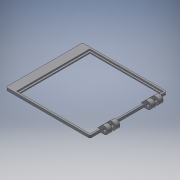
# Autodesk Inventor part: tampa acrilico
Saved by Autodesk Inventor 2019.4 (Build 234330000, 330)
## iProperties
Created: 2019-11-13
Part Number: tampa acrilico
Material: Genérico
Document SubType Name: Modeling
Designer: natha
Density: 1 g/cm^3
Appearance: Padrão
Author: natha
Autodesk Inventor part; units mm, degrees
ref_plane "YZ Plane" through (0, 0, 0) normal (1, 0, 0) x (0, 1, 0)
ref_plane "XZ Plane" through (0, 0, 0) normal (0, 1, 0) x (-1, 0, 0)
ref_plane "XY Plane" through (0, 0, 0) normal (0, 0, 1) x (1, 0, 0)
sketch "Esboço1" plane through (0, 0, 0) normal (0, 1, 0) x (-1, 0, 0)
  line L0 (-53, -48) -> (-53, 48)
  line L1 (-53, 48) -> (43, 48)
  line L2 (43, -48) -> (43, 48)
  line L3 (43, -48) -> (-53, -48)
  line L4 (-57, -52) -> (57, -52)
  line L5 (57, -52) -> (57, 52)
  line L6 (57, 52) -> (-57, 52)
  line L7 (-57, 52) -> (-57, 42.5)
  line L8 (-57, 42.5) -> (-57, 37.5)
  line L9 (-66.8204, 37.5) -> (-57, 37.5)
  line L10 (-66.8204, 31.9) -> (-66.8204, 37.5)
  line L11 (-66.8204, 31.9) -> (-57, 31.9)
  line L12 (-57, 31.9) -> (-57, 26.9)
  line L13 (-66.8204, 26.9) -> (-57, 26.9)
  line L14 (-66.8204, 21.3) -> (-66.8204, 26.9)
  line L15 (-66.8204, 21.3) -> (-57, 21.3)
  line L16 (-57, 21.3) -> (-57, 12.5)
  line L17 (-57, 12.5) -> (-57, -12.5)
  line L18 (-57, -12.5) -> (-57, -21.3)
  line L19 (-66.8204, -21.3) -> (-57, -21.3)
  line L20 (-66.8204, -26.9) -> (-66.8204, -21.3)
  line L21 (-66.8204, -26.9) -> (-57, -26.9)
  line L22 (-57, -26.9) -> (-57, -31.9)
  line L23 (-66.8204, -31.9) -> (-57, -31.9)
  line L24 (-66.8204, -37.5) -> (-66.8204, -31.9)
  line L25 (-66.8204, -37.5) -> (-57, -37.5)
  line L26 (-57, -37.5) -> (-57, -42.5)
  line L27 (-57, -42.5) -> (-57, -52)
  point P0 (0, 0)
  point P1 (0, 0)
  constraints: 56 end point
extrude "Extrusão1" add sketch "Esboço1" along normal blind 3.5
sketch "Esboço8" plane through (57, 0, 37.5) normal (0, 0, 1) x (1, 0, 0)
  arc A0 (6.3229, 3.5) -> (3.6771, 3.5) centre (5, 5) ccw projected
  circle A1 centre (5, 5) radius 2
  point P0 (-57, 0)
  constraints: 1 centre point, 1 coincident
extrude "Extrusão7" cut sketch "Esboço8" against normal blind 104
sketch "Esboço11" plane through (57, 0, 37.5) normal (0, 0, 1) x (1, 0, 0)
  circle A0 centre (5, 5) radius 2 projected
  arc A1 (5, 0) -> (10, 5) centre (5, 5) ccw
  arc A2 (9.7697, 3.5) -> (0, 5) centre (5, 5) ccw projected
  line L0 (10, 5) -> (10, 0)
  line L1 (10, 0) -> (5, 0)
  point P0 (-57, 0)
  constraints: 4 end point, 3 point on circle, 3 tangent, 1 centre point, 1 coincident, 1 vertical
extrude "Extrusão8" cut sketch "Esboço11" against normal blind 104 contours A1 L0 L1
sketch "Esboço12" plane through (57, 0, 37.5) normal (0, 0, 1) x (1, 0, 0)
  circle A0 centre (4.9996, 5.0611) radius 2
  arc A1 (9.9996, 5.0611) -> (1.5877, 8.7161) centre (4.9996, 5.0611) ccw
  line L0 (0, 0.0611) -> (0, 3.5)
  line L1 (0, 0.0611) -> (4.9996, 0.0611)
  arc A2 (4.9996, 0.0611) -> (9.9996, 5.0611) centre (4.9996, 5.0611) ccw
  line L2 (0, 3.5) -> (0, 0.0611)
  arc A3 (9.7697, 3.5) -> (9.9996, 5.0611) centre (5, 5) ccw
  line L3 (-4, 3.5) -> (0, 3.5)
  line L4 (-4, 0) -> (-4, 3.5)
  line L5 (-4, 0) -> (-4, 3.5)
  line L6 (-4, 3.5) -> (1.5877, 8.7161)
  line L7 (0, 3.5) -> (-4, 3.5)
  point P0 (-57, 0)
  dimension "d26" = 5
  constraints: 16 end point, 6 point on circle, 4 centre point, 2 tangent, 1 coincident, 1 horizontal, 1 perpendicular, 1 point on line, 1 vertical
  measures "d26" radius of A2
extrude "Extrusão9" add sketch "Esboço12" against normal blind 75
sketch "Esboço13" plane through (57, 0, 52) normal (1, 0, 0) x (0, 0, -1)
  line L0 (0, 0) -> (14.5, 0) projected
  line L1 (14.5, 0) -> (14.5, 3.5) projected
  line L2 (0, 3.5) -> (14.5, 3.5) projected
  line L3 (0, 0) -> (0, 3.5) projected
  line L4 (14.5, 3.5) -> (20.1, 3.5) projected
  line L5 (14.5, 0) -> (14.5, 3.5) projected
  line L6 (20.1, 0) -> (14.5, 0) projected
  line L7 (20.1, 3.5) -> (20.1, 0) projected
  line L8 (25.1, 0) -> (25.1, 3.5) projected
  line L9 (30.7, 0) -> (25.1, 0) projected
  line L10 (30.7, 3.5) -> (30.7, 0) projected
  line L11 (25.1, 3.5) -> (30.7, 3.5) projected
  line L12 (73.3, 0) -> (73.3, 3.5) projected
  line L13 (78.9, 0) -> (73.3, 0) projected
  line L14 (78.9, 3.5) -> (78.9, 0) projected
  line L15 (73.3, 3.5) -> (78.9, 3.5) projected
  line L16 (83.9, 0) -> (83.9, 3.5) projected
  line L17 (89.5, 0) -> (83.9, 0) projected
  line L18 (89.5, 3.5) -> (89.5, 0) projected
  line L19 (83.9, 3.5) -> (89.5, 3.5) projected
  line L20 (14.5, 10.0611) -> (89.5, 10.0611) projected
  line L21 (20.1, 0) -> (25.1, 0)
  line L22 (25.1, 0) -> (25.1, 10.0611)
  line L23 (25.1, 10.0611) -> (20.1, 10.0611)
  line L24 (20.1, 10.0611) -> (20.1, 0)
  line L25 (89.5, 0) -> (83.9, 0) projected
  line L26 (83.9, 0) -> (78.9, 0)
  line L27 (78.9, 0) -> (78.9, 10.0611)
  line L28 (78.9, 10.0611) -> (83.9, 10.0611)
  line L29 (83.9, 10.0611) -> (83.9, 0)
  line L30 (73.3, 0) -> (30.7, 0)
  line L31 (30.7, 0) -> (30.7, 10.0611)
  line L32 (30.7, 10.0611) -> (73.3, 10.0611)
  line L33 (73.3, 10.0611) -> (73.3, 0)
  point P0 (52, 0)
  constraints: 24 end point, 6 parallel, 3 horizontal, 3 perpendicular, 3 point on line
extrude "Extrusão10" cut sketch "Esboço13" along normal blind 10 contours L7 L24 L20 L22 L8 L21 | L10 L31 L20 L33 L12 L30 | L14 L27 L20 L29 L16 L26
sketch "Esboço15" plane through (57, 0, 21.3) normal (1, 0, 0) x (0, 0, -1)
  line L0 (-10.6, 0) -> (-10.6, 7.234)
  line L1 (-10.6, 0) -> (-5.6, 0)
  line L2 (-5.6, 7.234) -> (-5.6, 0)
  line L3 (-10.6, 7.234) -> (-5.6, 7.234)
  line L4 (0, 0) -> (0, 7.234)
  line L5 (0, 0) -> (42.6, 0)
  line L6 (42.6, 7.234) -> (42.6, 0)
  line L7 (0, 7.234) -> (42.6, 7.234)
  line L8 (-16.2, 3.5) -> (-10.6, 3.5)
  line L9 (-16.2, 0) -> (-16.2, 3.5)
  line L10 (-10.6, 0) -> (-16.2, 0)
  line L11 (-10.6, 3.5) -> (-10.6, 0)
  line L12 (-5.6, 0) -> (-5.6, 3.5)
  line L13 (0, 0) -> (-5.6, 0)
  line L14 (0, 3.5) -> (0, 0)
  line L15 (-5.6, 3.5) -> (0, 3.5)
  line L16 (-10.6, 3.5) -> (-5.6, 3.5)
  line L17 (-5.6, 3.5) -> (-5.6, 7.234)
  line L18 (-5.6, 7.234) -> (-10.6, 7.234)
  line L19 (-10.6, 7.234) -> (-10.6, 3.5)
  line L20 (48.2, 0) -> (48.2, 7.234)
  line L21 (48.2, 0) -> (53.2, 0)
  line L22 (53.2, 7.234) -> (53.2, 0)
  line L23 (48.2, 7.234) -> (53.2, 7.234)
  line L24 (42.6, 0) -> (42.6, 3.5)
  line L25 (48.2, 0) -> (42.6, 0)
  line L26 (48.2, 3.5) -> (48.2, 0)
  line L27 (42.6, 3.5) -> (48.2, 3.5)
  line L28 (53.2, 0) -> (53.2, 3.5)
  line L29 (58.8, 0) -> (53.2, 0)
  line L30 (58.8, 3.5) -> (58.8, 0)
  line L31 (53.2, 3.5) -> (58.8, 3.5)
  line L32 (53.2, 7.234) -> (48.2, 7.234)
  line L33 (48.2, 7.234) -> (48.2, 3.5)
  line L34 (48.2, 3.5) -> (53.2, 3.5)
  line L35 (53.2, 3.5) -> (53.2, 7.234)
  line L36 (42.6, 7.234) -> (0, 7.234)
  line L37 (0, 7.234) -> (0, 3.5)
  line L38 (0, 3.5) -> (42.6, 3.5)
  line L39 (42.6, 3.5) -> (42.6, 7.234)
  point P0 (21.3, 0)
extrude "Extrusão11" cut sketch "Esboço15" against normal blind 10 contours L0 L3 L2 L16 | L4 L7 L6 L38 | L20 L23 L22 L34
sketch "Esboço16" plane through (0, 3.5, 0) normal (0, 1, 0) x (1, 0, 0)
  line L0 (-43, 48) -> (53, 48) projected
  line L1 (53, -48) -> (-43, -48) projected
  line L2 (53, 21.3) -> (53, -21.3) projected
  line L3 (-43, -48) -> (-43, 48) projected
  line L4 (-43, -48) -> (-43, 0) construction
  line L5 (-43, 48) -> (-43, -48) construction
  line L6 (-43, 0) -> (5, 0) construction
  line L7 (55, -49.7497) -> (-45, -49.7497)
  line L8 (-45, -49.7497) -> (-45, 49.7497)
  line L9 (-45, 49.7497) -> (55, 49.7497)
  line L10 (55, 49.7497) -> (55, -49.7497)
  line L11 (55, -49.7497) -> (-45, 49.7497) construction
  line L12 (-45, -49.7497) -> (55, 49.7497) construction
  point P0 (0, 0)
  dimension "d33" = 96
  dimension "d34" = 96
  dimension "d35" = 48
  dimension "d36" = 100
  constraints: 16 end point, 3 midpoint, 2 horizontal, 2 parallel, 1 perpendicular
  measures "d33" distance between parallel lines of L0 L1
  measures "d34" distance between parallel lines of L2 L3
  measures "d35" distance of L4.end L6.end
  measures "d36" distance of L8.end L9.end
extrude "Extrusão12" cut sketch "Esboço16" against normal blind 2
fillet "Arredondamento1" radius 2 4 edges at (57, 1.75, 52) (57, 1.75, -52) (-57, 1.75, -52) (-57, 1.75, 52)
